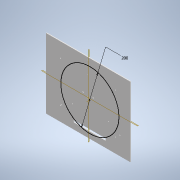
# Autodesk Inventor part: панель_электроники_и не только
Saved by Autodesk Inventor 2021.1 (Build 251245010, 245A)
## iProperties
Created: 2022-11-16
Part Number: панель_электроники_и не только
Material: Типовые
Document SubType Name: Modeling
Designer: zmoze
Density: 1 g/cm^3
Appearance: По умолчанию
Author: zmoze
Autodesk Inventor part; units mm, degrees
ref_plane "YZ Plane" through (0, 0, 0) normal (1, 0, 0) x (0, 1, 0)
ref_plane "XZ Plane" through (0, 0, 0) normal (0, 1, 0) x (-1, 0, 0)
ref_plane "XY Plane" through (0, 0, 0) normal (0, 0, 1) x (1, 0, 0)
sketch "Эскиз1" plane through (0, 0, 0) normal (0, 0, 1) x (1, 0, 0)
  line L0 (-150.6635, -115.8017) -> (139.3365, -115.8017)
  line L1 (139.3365, -115.8017) -> (139.3365, 124.1983)
  line L2 (139.3365, 124.1983) -> (-150.6635, 124.1983)
  line L3 (-150.6635, 124.1983) -> (-150.6635, -115.8017)
  line L4 (139.3365, -115.8017) -> (-150.6635, 124.1983) construction
  line L5 (-150.6635, -115.8017) -> (139.3365, 124.1983) construction
  point P0 (-5.6635, 4.1983)
  point P1 (-5.6635, 4.1983)
  point P2 (-5.6635, 4.1983)
  dimension "d0" = 240
  dimension "d1" = 290
  constraints: 12 end point, 2 coincident, 2 midpoint, 2 parallel, 1 horizontal, 1 perpendicular
  measures "d0" distance of L2.end L0.start
  measures "d1" distance of L1.end L2.end
extrude "Выдавливание1" add sketch "Эскиз1" along normal blind 3
sketch "Эскиз2" plane through (0, 0, 3) normal (0, 0, 1) x (1, 0, 0)
  circle A0 centre (0, 0) radius 100
  dimension "d4" = 200
  constraints: 1 centre point, 1 coincident
  measures "d4" diameter of A0
ref_plane "РабПлоскость1" through (-5.6635, -115.8017, 0) normal (-1, 0, 0) x (0, 0, 1)
ref_plane "РабПлоскость2" through (-150.6635, 4.1983, 0) normal (0, 1, 0) x (1, 0, 0)
sketch "Эскиз3" plane through (0, 0, 3) normal (0, 0, 1) x (1, 0, 0)
  circle A0 centre (-97.799, -63.0039) radius 1.5 projected
  circle A1 centre (-59.6938, -41.0039) radius 1.5 projected
  circle A2 centre (103.4624, -53.1945) radius 1.5 projected
  circle A3 centre (65.3573, -31.1945) radius 1.5 projected
  circle A4 centre (-5.6635, 72.1983) radius 1.5 projected
  circle A5 centre (-5.6635, 116.1983) radius 1.5 projected
  point P0 (0, 0)
extrude "Выдавливание2" cut sketch "Эскиз3" against normal blind 10
sketch "Эскиз4" plane through (0, 0, 0) normal (0, 0, -1) x (-1, 0, 0)
  line L0 (-55, -94.3017) -> (55, -94.3017)
  line L1 (55, -94.3017) -> (55, -87.3017)
  line L2 (55, -87.3017) -> (-55, -87.3017)
  line L3 (-55, -87.3017) -> (-55, -94.3017)
  line L4 (0, 0) -> (0, 37.9821) construction
  line L5 (150.6635, -115.8017) -> (-139.3365, -115.8017) construction
  line L6 (-11.6132, -94.8017) -> (-38.9526, -94.8017) projected
  line L7 (-11.6132, -89.8017) -> (-38.9526, -89.8017) projected
  point P0 (0, -87.3017)
  dimension "d7" = 7
  dimension "d8" = 55
  dimension "d9" = 21.5
  constraints: 10 end point, 2 parallel, 1 horizontal, 1 midpoint, 1 perpendicular, 1 point on line, 1 vertical
  measures "d7" distance between parallel lines of L2 L0
  measures "d8" horizontal distance of L4.start L0.start
  measures "d9" distance between parallel lines of L5 L0
extrude "Выдавливание3" cut sketch "Эскиз4" against normal blind 10
sketch "Эскиз6" plane through (0, 0, 3) normal (0, 0, 1) x (1, 0, 0)
  circle A0 centre (-23.1635, 12.1983) radius 2 projected
  circle A1 centre (11.8365, 12.1983) radius 2 projected
  line L0 (55, -87.3017) -> (-55, -87.3017) projected
  line L1 (-55, -87.3017) -> (-55, -94.3017) projected
  line L2 (-55, -94.3017) -> (55, -94.3017) projected
  line L3 (55, -94.3017) -> (55, -87.3017) projected
  circle A2 centre (65.3573, -31.1945) radius 1.5 projected
  circle A3 centre (-97.799, -63.0039) radius 1.5 projected
  circle A4 centre (103.4624, -53.1945) radius 1.5 projected
  circle A5 centre (-59.6938, -41.0039) radius 1.5 projected
  circle A6 centre (-5.6635, 72.1983) radius 1.5 projected
  circle A7 centre (-5.6635, 116.1983) radius 1.5 projected
  line L4 (139.3365, -115.8017) -> (139.3365, 124.1983) projected
  line L5 (-150.6635, -115.8017) -> (139.3365, -115.8017) projected
  line L6 (-150.6635, 124.1983) -> (-150.6635, -115.8017) projected
  line L7 (139.3365, 124.1983) -> (-150.6635, 124.1983) projected
  arc A8 (-7.1635, 6.1983) -> (-7.1635, 2.1983) centre (-5.6635, 4.1983) ccw projected
  circle A9 centre (-5.6635, 4.1983) radius 2.6
  point P0 (0, 0)
  point P1 (0.9551, 9.8906)
  dimension "d16" = 0.1
  constraints: 1 centre point, 1 coincident, 1 other
  measures "d16" radial gap between concentric circles of A9 A8
extrude "Выдавливание5" cut sketch "Эскиз6" against normal blind 10 contours A0 | A1 | A9
sketch "Эскиз7" plane through (0, 0, 3) normal (0, 0, 1) x (1, 0, 0)
  circle A0 centre (89.3365, -75.8017) radius 1.5 projected
  circle A1 centre (89.3365, 84.1983) radius 1.5 projected
  circle A2 centre (-100.6635, 84.1983) radius 1.5 projected
  line L0 (-150.6635, -115.8017) -> (139.3365, -115.8017) projected
  line L1 (-150.6635, 124.1983) -> (-150.6635, -115.8017) projected
  circle A3 centre (-100.6635, -75.8017) radius 1.5 projected
  point P0 (0, 0)
extrude "Выдавливание6" cut sketch "Эскиз7" against normal blind 10
